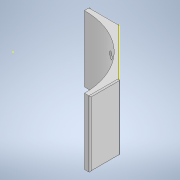
# Autodesk Inventor part: refuerzo brazo
Saved by Autodesk Inventor 2021 (Build 250183000, 183)
## iProperties
Created: 2021-03-15
Part Number: refuerzo brazo
Material: Genérico
Document SubType Name: Modeling
Designer: Joaquín
Density: 1 g/cm^3
Appearance: Valor por defecto
Author: Joaquín
Autodesk Inventor part; units mm, degrees
ref_plane "YZ Plane" through (0, 0, 0) normal (1, 0, 0) x (0, 1, 0)
ref_plane "XZ Plane" through (0, 0, 0) normal (0, 1, 0) x (-1, 0, 0)
ref_plane "XY Plane" through (0, 0, 0) normal (0, 0, 1) x (1, 0, 0)
sketch "Boceto1" plane through (0, 0, 0) normal (0, 1, 0) x (-1, 0, 0)
  arc A0 (-32.5, 0) -> (0, -32.5) centre (0, 0) ccw
  line L0 (-32.5, 0) -> (-35, 0)
  line L1 (0, -32.5) -> (0, -35)
  line L2 (-35, 0) -> (-35, -13.4629)
  line L3 (0, -35) -> (-13.4629, -35)
  line L4 (-35, -13.4629) -> (-13.4629, -35)
  dimension "d2" = 2.5
  dimension "d3" = 2.5
  constraints: 10 end point, 2 point on circle, 2 vertical, 1 centre point, 1 coincident, 1 horizontal, 1 perpendicular
  measures "d2" distance of L0.start L0.end
  measures "d3" distance of L1.start L1.end
extrude "Extrusión1" add sketch "Boceto1" along normal blind 30
sketch "Boceto2" plane through (0, 30, 0) normal (0, 1, 0) x (1, 0, 0)
  line L0 (35, 13.4629) -> (13.4629, 35) projected
  point P0 (0, 0)
fillet "Empalme1" radius 0.5 10 edges at (35, 30, -6.7315) (24.2315, 30, -24.2315) (35, 15, -13.4629) (24.2315, 0, -24.2315) (35, 0, -6.7315) (13.4629, 15, -35) (6.7315, 30, -35) (0, 15, -35) (6.7315, 0, -35) (35, 15, 0)
sketch "Boceto9" plane through (13.6094, 0.5, -34.8536) normal (0.7071, 0, -0.7071) x (-0.7071, 0, -0.7071)
  line L0 (-29.1913, 16.5896) -> (-13.5718, 16.5896) construction
  line L1 (-13.5718, 16.5896) -> (-13.5718, 13.5396) construction
  line L2 (-13.5718, 13.5396) -> (-29.1913, 13.5396) construction
  line L3 (-29.1913, 13.5396) -> (-29.1913, 16.5896) construction
  line L4 (-24.9703, 16.5896) -> (-24.9703, 14.2431)
  line L5 (-24.9703, 14.2431) -> (-24.0308, 14.2431)
  spline S0 degree 2 poles (-24.0308, 14.2431) (-23.8337, 14.2385) (-23.561, 14.3806) (-23.561, 14.4745) knots 0 0 0 1 2 2 2
  line L6 (-23.561, 14.4745) -> (-23.561, 16.5896)
  line L7 (-23.561, 16.5896) -> (-22.1541, 16.5896)
  line L8 (-22.1541, 16.5896) -> (-22.1541, 14.4791)
  spline S1 degree 2 poles (-22.1541, 14.4791) (-22.1541, 14.0895) (-23.2517, 13.5396) (-24.0308, 13.5396) knots 0 0 0 1 2 2 2
  line L9 (-24.0308, 13.5396) -> (-27.3145, 13.5396)
  spline S2 degree 2 poles (-27.3145, 13.5396) (-28.0845, 13.5396) (-29.1913, 14.0895) (-29.1913, 14.4722) knots 0 0 0 1 2 2 2
  line L10 (-29.1913, 14.4722) -> (-29.1913, 16.5896)
  line L11 (-29.1913, 16.5896) -> (-27.7843, 16.5896)
  line L12 (-27.7843, 16.5896) -> (-27.7843, 14.4814)
  spline S3 degree 2 poles (-27.7843, 14.4814) (-27.7843, 14.3897) (-27.5208, 14.2568) (-27.3627, 14.2431) knots 0 0 0 1 2 2 2
  spline S4 degree 2 poles (-27.3627, 14.2431) (-27.3535, 14.2431) (-27.3237, 14.2431) (-27.3145, 14.2431) knots 0 0 0 1 2 2 2
  line L13 (-27.3145, 14.2431) -> (-26.3773, 14.2431)
  line L14 (-26.3773, 14.2431) -> (-26.3773, 16.5896)
  line L15 (-26.3773, 16.5896) -> (-24.9703, 16.5896)
  line L16 (-20.2773, 13.5396) -> (-21.6843, 13.5396)
  line L17 (-21.6843, 13.5396) -> (-21.6843, 16.5896)
  line L18 (-21.6843, 16.5896) -> (-20.2773, 16.5896)
  line L19 (-20.2773, 16.5896) -> (-20.2773, 13.5396)
  line L20 (-14.1796, 13.5396) -> (-17.9308, 13.5396)
  spline S5 degree 2 poles (-17.9308, 13.5396) (-18.7008, 13.5396) (-19.8076, 14.0895) (-19.8076, 14.4722) knots 0 0 0 1 2 2 2
  line L21 (-19.8076, 14.4722) -> (-19.8076, 16.5896)
  line L22 (-19.8076, 16.5896) -> (-18.4006, 16.5896)
  line L23 (-18.4006, 16.5896) -> (-18.4006, 14.4791)
  spline S6 degree 2 poles (-18.4006, 14.4791) (-18.4006, 14.3806) (-18.1187, 14.2385) (-17.9308, 14.2385) knots 0 0 0 1 2 2 2
  line L24 (-17.9308, 14.2385) -> (-14.1796, 14.2385)
  line L25 (-14.1796, 14.2385) -> (-14.1796, 13.5396)
  line L26 (-8.0819, 13.5396) -> (-11.8331, 13.5396)
  spline S7 degree 2 poles (-11.8331, 13.5396) (-12.603, 13.5396) (-13.7098, 14.0895) (-13.7098, 14.4722) knots 0 0 0 1 2 2 2
  line L27 (-13.7098, 14.4722) -> (-13.7098, 16.5896)
  line L28 (-13.7098, 16.5896) -> (-12.3029, 16.5896)
  line L29 (-12.3029, 16.5896) -> (-12.3029, 14.4791)
  spline S8 degree 2 poles (-12.3029, 14.4791) (-12.3029, 14.3806) (-12.021, 14.2385) (-11.8331, 14.2385) knots 0 0 0 1 2 2 2
  line L30 (-11.8331, 14.2385) -> (-8.0819, 14.2385)
  line L31 (-8.0819, 14.2385) -> (-8.0819, 13.5396)
  line L32 (-3.3912, 13.5396) -> (-4.7982, 13.5396)
  line L33 (-4.7982, 13.5396) -> (-4.7982, 14.7128)
  line L34 (-4.7982, 14.7128) -> (-5.7354, 14.7128)
  spline S9 degree 2 poles (-5.7354, 14.7128) (-6.5053, 14.7082) (-7.6121, 15.2628) (-7.6121, 15.6455) knots 0 0 0 1 2 2 2
  line L35 (-7.6121, 15.6455) -> (-7.6121, 16.5896)
  line L36 (-7.6121, 16.5896) -> (-6.2051, 16.5896)
  line L37 (-6.2051, 16.5896) -> (-6.2051, 15.6523)
  spline S10 degree 2 poles (-6.2051, 15.6523) (-6.2051, 15.5584) (-5.9416, 15.4255) (-5.7835, 15.4117) knots 0 0 0 1 2 2 2
  spline S11 degree 2 poles (-5.7835, 15.4117) (-5.7743, 15.4117) (-5.7446, 15.4117) (-5.7354, 15.4117) knots 0 0 0 1 2 2 2
  line L38 (-5.7354, 15.4117) -> (-2.4517, 15.4117)
  spline S12 degree 2 poles (-2.4517, 15.4117) (-2.2546, 15.4071) (-1.9819, 15.5492) (-1.9819, 15.6432) knots 0 0 0 1 2 2 2
  line L39 (-1.9819, 15.6432) -> (-1.9819, 16.5896)
  line L40 (-1.9819, 16.5896) -> (-0.5749, 16.5896)
  line L41 (-0.5749, 16.5896) -> (-0.5749, 15.6546)
  spline S13 degree 2 poles (-0.5749, 15.6546) (-0.5749, 15.2651) (-1.6725, 14.7128) (-2.4517, 14.7128) knots 0 0 0 1 2 2 2
  line L42 (-2.4517, 14.7128) -> (-3.3912, 14.7128)
  line L43 (-3.3912, 14.7128) -> (-3.3912, 13.5396)
  point P0 (-15.0219, -0.5)
  constraints: 2 other
extrude "Extrusión3" cut sketch "Boceto9" against normal blind 1
sketch "Boceto11" plane through (13.6094, 0.5, -34.8536) normal (0.7071, 0, -0.7071) x (-0.7071, 0, -0.7071)
  line L0 (-38.0029, 29.5) -> (7.9591, 29.5) projected
  circle A0 centre (-23.0219, 22.5) radius 1.5
  circle A1 centre (-7.0219, 22.5) radius 1.5
  circle A2 centre (-7.0219, 6.5) radius 1.5
  circle A3 centre (-23.0219, 6.5) radius 1.5
  point P0 (-15.0219, -0.5)
  constraints: 4 centre point
extrude "Extrusión4" cut sketch "Boceto11" along normal mid plane 10
